Autodesk Fusion 360 part; units mm, degrees
(part 5 of 6)
  line L2682 (181.3394, 91.625) -> (181.127, 93.125)
  line L2683 (187.1203, 93.125) -> (188.1063, 86.1615)
  line L2684 (181.3454, 86.0752) -> (182.0837, 85.3126)
  line L2685 (180.927, 93.125) -> (181.8208, 86.8124)
  line L2686 (187.186, 86.0499) -> (186.4477, 86.8126)
  line L2687 (186.4603, 87.0871) -> (185.6054, 93.125)
  line L2688 (181.127, 93.125) -> (185.4054, 93.125)
  line L2689 (186.4477, 86.8126) -> (182.1089, 86.8126)
  line L2690 (185.6054, 93.125) -> (187.1203, 93.125)
  line L2691 (181.8208, 86.8124) -> (181.1478, 86.1625)
  line L2692 (198.3258, 91.625) -> (194.0474, 91.625)
  line L2693 (193.635, 93.125) -> (192.12, 93.125)
  arc A395 (201.2525, 79) -> (201.7476, 79.5701) centre (201.2525, 79.5) ccw
  circle A396 centre (192.12, 79.875) radius 0.875
  line L2694 (193.8842, 85.9625) -> (194.7802, 85.0369)
  line L2695 (200.3283, 79) -> (201.8283, 79)
  line L2696 (199.9139, 80.5) -> (195.6246, 80.5)
  line L2697 (194.8169, 86.8126) -> (194.0534, 86.0752)
  line L2698 (195.635, 79) -> (194.12, 79)
  line L2699 (194.12, 79) -> (193.1342, 85.9625)
  line L2700 (199.4326, 85.3263) -> (200.3283, 79)
  line L2701 (200.1263, 79) -> (199.9139, 80.5)
  line L2702 (199.1304, 85.3126) -> (199.894, 86.0499)
  line L2703 (200.8143, 86.1615) -> (200.0643, 86.1615)
  line L2704 (201.8283, 79) -> (200.8424, 85.9635)
  arc A397 (192.6958, 93.125) -> (192.2007, 92.5549) centre (192.6958, 92.625) ccw
  line L2705 (195.837, 79) -> (200.1263, 79)
  line L2706 (194.7802, 85.0369) -> (195.635, 79)
  line L2707 (200.0924, 85.9635) -> (199.4326, 85.3263)
  line L2708 (195.6246, 80.5) -> (195.837, 79)
  line L2709 (194.7917, 85.3126) -> (199.1304, 85.3126)
  line L2710 (200.0643, 86.1615) -> (199.1683, 87.0871)
  line L2711 (193.1342, 85.9625) -> (193.8842, 85.9625)
  line L2712 (200.8424, 85.9635) -> (200.0924, 85.9635)
  arc A398 (194.0591, 79.4299) -> (194.5542, 79) centre (194.5542, 79.5) ccw
  line L2713 (193.8558, 86.1625) -> (193.1058, 86.1625)
  line L2714 (198.1134, 93.125) -> (198.3258, 91.625)
  arc A399 (199.8892, 92.6951) -> (199.3941, 93.125) centre (199.3941, 92.625) ccw
  line L2715 (193.1058, 86.1625) -> (192.12, 93.125)
  line L2716 (194.0474, 91.625) -> (193.835, 93.125)
  line L2717 (199.8283, 93.125) -> (200.8143, 86.1615)
  line L2718 (194.0534, 86.0752) -> (194.7917, 85.3126)
  line L2719 (193.635, 93.125) -> (194.5288, 86.8124)
  line L2720 (199.894, 86.0499) -> (199.1557, 86.8126)
  line L2721 (199.1683, 87.0871) -> (198.3134, 93.125)
  line L2722 (193.835, 93.125) -> (198.1134, 93.125)
  line L2723 (199.1557, 86.8126) -> (194.8169, 86.8126)
  line L2724 (198.3134, 93.125) -> (199.8283, 93.125)
  line L2725 (194.5288, 86.8124) -> (193.8558, 86.1625)
  line L2726 (7.7058, 110.75) -> (3.4274, 110.75)
  line L2727 (3.015, 112.25) -> (1.5, 112.25)
  arc A400 (10.6325, 98.125) -> (11.1276, 98.6951) centre (10.6325, 98.625) ccw
  circle A401 centre (1.5, 99) radius 0.875
  line L2728 (3.2642, 105.0875) -> (4.1602, 104.1619)
  line L2729 (9.7083, 98.125) -> (11.2083, 98.125)
  line L2730 (9.2939, 99.625) -> (5.0046, 99.625)
  line L2731 (4.1969, 105.9376) -> (3.4334, 105.2002)
  line L2732 (5.015, 98.125) -> (3.5, 98.125)
  line L2733 (3.5, 98.125) -> (2.5142, 105.0875)
  line L2734 (8.8126, 104.4513) -> (9.7083, 98.125)
  line L2735 (9.5063, 98.125) -> (9.2939, 99.625)
  line L2736 (8.5104, 104.4376) -> (9.274, 105.1749)
  line L2737 (10.1943, 105.2865) -> (9.4443, 105.2865)
  line L2738 (11.2083, 98.125) -> (10.2224, 105.0885)
  arc A402 (2.0758, 112.25) -> (1.5807, 111.6799) centre (2.0758, 111.75) ccw
  line L2739 (5.217, 98.125) -> (9.5063, 98.125)
  line L2740 (4.1602, 104.1619) -> (5.015, 98.125)
  line L2741 (9.4724, 105.0885) -> (8.8126, 104.4513)
  line L2742 (5.0046, 99.625) -> (5.217, 98.125)
  line L2743 (4.1717, 104.4376) -> (8.5104, 104.4376)
  line L2744 (9.4443, 105.2865) -> (8.5483, 106.2121)
  line L2745 (2.5142, 105.0875) -> (3.2642, 105.0875)
  line L2746 (10.2224, 105.0885) -> (9.4724, 105.0885)
  arc A403 (3.4391, 98.5549) -> (3.9342, 98.125) centre (3.9342, 98.625) ccw
  line L2747 (3.2358, 105.2875) -> (2.4858, 105.2875)
  line L2748 (7.4934, 112.25) -> (7.7058, 110.75)
  arc A404 (9.2692, 111.8201) -> (8.7741, 112.25) centre (8.7741, 111.75) ccw
  line L2749 (2.4858, 105.2875) -> (1.5, 112.25)
  line L2750 (3.4274, 110.75) -> (3.215, 112.25)
  line L2751 (9.2083, 112.25) -> (10.1943, 105.2865)
  line L2752 (3.4334, 105.2002) -> (4.1717, 104.4376)
  line L2753 (3.015, 112.25) -> (3.9088, 105.9374)
  line L2754 (9.274, 105.1749) -> (8.5357, 105.9376)
  line L2755 (8.5483, 106.2121) -> (7.6934, 112.25)
  line L2756 (3.215, 112.25) -> (7.4934, 112.25)
  line L2757 (8.5357, 105.9376) -> (4.1969, 105.9376)
  line L2758 (7.6934, 112.25) -> (9.2083, 112.25)
  line L2759 (3.9088, 105.9374) -> (3.2358, 105.2875)
  line L2760 (20.4138, 110.75) -> (16.1354, 110.75)
  line L2761 (15.723, 112.25) -> (14.208, 112.25)
  arc A405 (23.3405, 98.125) -> (23.8356, 98.6951) centre (23.3405, 98.625) ccw
  circle A406 centre (14.208, 99) radius 0.875
  line L2762 (15.9722, 105.0875) -> (16.8682, 104.1619)
  line L2763 (22.4163, 98.125) -> (23.9163, 98.125)
  line L2764 (22.0019, 99.625) -> (17.7126, 99.625)
  line L2765 (16.9049, 105.9376) -> (16.1414, 105.2002)
  line L2766 (17.723, 98.125) -> (16.208, 98.125)
  line L2767 (16.208, 98.125) -> (15.2222, 105.0875)
  line L2768 (21.5206, 104.4513) -> (22.4163, 98.125)
  line L2769 (22.2143, 98.125) -> (22.0019, 99.625)
  line L2770 (21.2184, 104.4376) -> (21.982, 105.1749)
  line L2771 (22.9023, 105.2865) -> (22.1523, 105.2865)
  line L2772 (23.9163, 98.125) -> (22.9304, 105.0885)
  arc A407 (14.7838, 112.25) -> (14.2887, 111.6799) centre (14.7838, 111.75) ccw
  line L2773 (17.925, 98.125) -> (22.2143, 98.125)
  line L2774 (16.8682, 104.1619) -> (17.723, 98.125)
  line L2775 (22.1804, 105.0885) -> (21.5206, 104.4513)
  line L2776 (17.7126, 99.625) -> (17.925, 98.125)
  line L2777 (16.8797, 104.4376) -> (21.2184, 104.4376)
  line L2778 (22.1523, 105.2865) -> (21.2563, 106.2121)
  line L2779 (15.2222, 105.0875) -> (15.9722, 105.0875)
  line L2780 (22.9304, 105.0885) -> (22.1804, 105.0885)
  arc A408 (16.1471, 98.5549) -> (16.6422, 98.125) centre (16.6422, 98.625) ccw
  line L2781 (15.9438, 105.2875) -> (15.1938, 105.2875)
  line L2782 (20.2014, 112.25) -> (20.4138, 110.75)
  arc A409 (21.9772, 111.8201) -> (21.4821, 112.25) centre (21.4821, 111.75) ccw
  line L2783 (15.1938, 105.2875) -> (14.208, 112.25)
  line L2784 (16.1354, 110.75) -> (15.923, 112.25)
  line L2785 (21.9163, 112.25) -> (22.9023, 105.2865)
  line L2786 (16.1414, 105.2002) -> (16.8797, 104.4376)
  line L2787 (15.723, 112.25) -> (16.6168, 105.9374)
  line L2788 (21.982, 105.1749) -> (21.2437, 105.9376)
  line L2789 (21.2563, 106.2121) -> (20.4014, 112.25)
  line L2790 (15.923, 112.25) -> (20.2014, 112.25)
  line L2791 (21.2437, 105.9376) -> (16.9049, 105.9376)
  line L2792 (20.4014, 112.25) -> (21.9163, 112.25)
  line L2793 (16.6168, 105.9374) -> (15.9438, 105.2875)
  line L2794 (33.1218, 110.75) -> (28.8434, 110.75)
  line L2795 (28.431, 112.25) -> (26.916, 112.25)
  arc A410 (36.0485, 98.125) -> (36.5436, 98.6951) centre (36.0485, 98.625) ccw
  circle A411 centre (26.916, 99) radius 0.875
  line L2796 (28.6802, 105.0875) -> (29.5762, 104.1619)
  line L2797 (35.1243, 98.125) -> (36.6243, 98.125)
  line L2798 (34.7099, 99.625) -> (30.4206, 99.625)
  line L2799 (29.6129, 105.9376) -> (28.8494, 105.2002)
  line L2800 (30.431, 98.125) -> (28.916, 98.125)
  line L2801 (28.916, 98.125) -> (27.9302, 105.0875)
  line L2802 (34.2286, 104.4513) -> (35.1243, 98.125)
  line L2803 (34.9223, 98.125) -> (34.7099, 99.625)
  line L2804 (33.9264, 104.4376) -> (34.69, 105.1749)
  line L2805 (35.6103, 105.2865) -> (34.8603, 105.2865)
  line L2806 (36.6243, 98.125) -> (35.6384, 105.0885)
  arc A412 (27.4918, 112.25) -> (26.9967, 111.6799) centre (27.4918, 111.75) ccw
  line L2807 (30.633, 98.125) -> (34.9223, 98.125)
  line L2808 (29.5762, 104.1619) -> (30.431, 98.125)
  line L2809 (34.8884, 105.0885) -> (34.2286, 104.4513)
  line L2810 (30.4206, 99.625) -> (30.633, 98.125)
  line L2811 (29.5877, 104.4376) -> (33.9264, 104.4376)
  line L2812 (34.8603, 105.2865) -> (33.9643, 106.2121)
  line L2813 (27.9302, 105.0875) -> (28.6802, 105.0875)
  line L2814 (35.6384, 105.0885) -> (34.8884, 105.0885)
  arc A413 (28.8551, 98.5549) -> (29.3502, 98.125) centre (29.3502, 98.625) ccw
  line L2815 (28.6518, 105.2875) -> (27.9018, 105.2875)
  line L2816 (32.9094, 112.25) -> (33.1218, 110.75)
  arc A414 (34.6852, 111.8201) -> (34.1901, 112.25) centre (34.1901, 111.75) ccw
  line L2817 (27.9018, 105.2875) -> (26.916, 112.25)
  line L2818 (28.8434, 110.75) -> (28.631, 112.25)
  line L2819 (34.6243, 112.25) -> (35.6103, 105.2865)
  line L2820 (28.8494, 105.2002) -> (29.5877, 104.4376)
  line L2821 (28.431, 112.25) -> (29.3248, 105.9374)
  line L2822 (34.69, 105.1749) -> (33.9517, 105.9376)
  line L2823 (33.9643, 106.2121) -> (33.1094, 112.25)
  line L2824 (28.631, 112.25) -> (32.9094, 112.25)
  line L2825 (33.9517, 105.9376) -> (29.6129, 105.9376)
  line L2826 (33.1094, 112.25) -> (34.6243, 112.25)
  line L2827 (29.3248, 105.9374) -> (28.6518, 105.2875)
  line L2828 (45.8298, 110.75) -> (41.5514, 110.75)
  line L2829 (41.139, 112.25) -> (39.624, 112.25)
  arc A415 (48.7565, 98.125) -> (49.2516, 98.6951) centre (48.7565, 98.625) ccw
  circle A416 centre (39.624, 99) radius 0.875
  line L2830 (41.3882, 105.0875) -> (42.2842, 104.1619)
  line L2831 (47.8323, 98.125) -> (49.3323, 98.125)
  line L2832 (47.4179, 99.625) -> (43.1286, 99.625)
  line L2833 (42.3209, 105.9376) -> (41.5574, 105.2002)
  line L2834 (43.139, 98.125) -> (41.624, 98.125)
  line L2835 (41.624, 98.125) -> (40.6382, 105.0875)
  line L2836 (46.9366, 104.4513) -> (47.8323, 98.125)
  line L2837 (47.6303, 98.125) -> (47.4179, 99.625)
  line L2838 (46.6344, 104.4376) -> (47.398, 105.1749)
  line L2839 (48.3183, 105.2865) -> (47.5683, 105.2865)
  line L2840 (49.3323, 98.125) -> (48.3464, 105.0885)
  arc A417 (40.1998, 112.25) -> (39.7047, 111.6799) centre (40.1998, 111.75) ccw
  line L2841 (43.341, 98.125) -> (47.6303, 98.125)
  line L2842 (42.2842, 104.1619) -> (43.139, 98.125)
  line L2843 (47.5964, 105.0885) -> (46.9366, 104.4513)
  line L2844 (43.1286, 99.625) -> (43.341, 98.125)
  line L2845 (42.2957, 104.4376) -> (46.6344, 104.4376)
  line L2846 (47.5683, 105.2865) -> (46.6723, 106.2121)
  line L2847 (40.6382, 105.0875) -> (41.3882, 105.0875)
  line L2848 (48.3464, 105.0885) -> (47.5964, 105.0885)
  arc A418 (41.5631, 98.5549) -> (42.0582, 98.125) centre (42.0582, 98.625) ccw
  line L2849 (41.3598, 105.2875) -> (40.6098, 105.2875)
  line L2850 (45.6174, 112.25) -> (45.8298, 110.75)
  arc A419 (47.3932, 111.8201) -> (46.8981, 112.25) centre (46.8981, 111.75) ccw
  line L2851 (40.6098, 105.2875) -> (39.624, 112.25)
  line L2852 (41.5514, 110.75) -> (41.339, 112.25)
  line L2853 (47.3323, 112.25) -> (48.3183, 105.2865)
  line L2854 (41.5574, 105.2002) -> (42.2957, 104.4376)
  line L2855 (41.139, 112.25) -> (42.0328, 105.9374)
  line L2856 (47.398, 105.1749) -> (46.6597, 105.9376)
  line L2857 (46.6723, 106.2121) -> (45.8174, 112.25)
  line L2858 (41.339, 112.25) -> (45.6174, 112.25)
  line L2859 (46.6597, 105.9376) -> (42.3209, 105.9376)
  line L2860 (45.8174, 112.25) -> (47.3323, 112.25)
  line L2861 (42.0328, 105.9374) -> (41.3598, 105.2875)
  line L2862 (58.5378, 110.75) -> (54.2594, 110.75)
  line L2863 (53.847, 112.25) -> (52.332, 112.25)
  arc A420 (61.4645, 98.125) -> (61.9596, 98.6951) centre (61.4645, 98.625) ccw
  circle A421 centre (52.332, 99) radius 0.875
  line L2864 (54.0962, 105.0875) -> (54.9922, 104.1619)
  line L2865 (60.5403, 98.125) -> (62.0403, 98.125)
  line L2866 (60.1259, 99.625) -> (55.8366, 99.625)
  line L2867 (55.0289, 105.9376) -> (54.2654, 105.2002)
  line L2868 (55.847, 98.125) -> (54.332, 98.125)
  line L2869 (54.332, 98.125) -> (53.3462, 105.0875)
  line L2870 (59.6446, 104.4513) -> (60.5403, 98.125)
  line L2871 (60.3383, 98.125) -> (60.1259, 99.625)
  line L2872 (59.3424, 104.4376) -> (60.106, 105.1749)
  line L2873 (61.0263, 105.2865) -> (60.2763, 105.2865)
  line L2874 (62.0403, 98.125) -> (61.0544, 105.0885)
  arc A422 (52.9078, 112.25) -> (52.4127, 111.6799) centre (52.9078, 111.75) ccw
  line L2875 (56.049, 98.125) -> (60.3383, 98.125)
  line L2876 (54.9922, 104.1619) -> (55.847, 98.125)
  line L2877 (60.3044, 105.0885) -> (59.6446, 104.4513)
  line L2878 (55.8366, 99.625) -> (56.049, 98.125)
  line L2879 (55.0037, 104.4376) -> (59.3424, 104.4376)
  line L2880 (60.2763, 105.2865) -> (59.3803, 106.2121)
  line L2881 (53.3462, 105.0875) -> (54.0962, 105.0875)
  line L2882 (61.0544, 105.0885) -> (60.3044, 105.0885)
  arc A423 (54.2711, 98.5549) -> (54.7662, 98.125) centre (54.7662, 98.625) ccw
  line L2883 (54.0678, 105.2875) -> (53.3178, 105.2875)
  line L2884 (58.3254, 112.25) -> (58.5378, 110.75)
  arc A424 (60.1012, 111.8201) -> (59.6061, 112.25) centre (59.6061, 111.75) ccw
  line L2885 (53.3178, 105.2875) -> (52.332, 112.25)
  line L2886 (54.2594, 110.75) -> (54.047, 112.25)
  line L2887 (60.0403, 112.25) -> (61.0263, 105.2865)
  line L2888 (54.2654, 105.2002) -> (55.0037, 104.4376)
  line L2889 (53.847, 112.25) -> (54.7408, 105.9374)
  line L2890 (60.106, 105.1749) -> (59.3677, 105.9376)
  line L2891 (59.3803, 106.2121) -> (58.5254, 112.25)
  line L2892 (54.047, 112.25) -> (58.3254, 112.25)
  line L2893 (59.3677, 105.9376) -> (55.0289, 105.9376)
  line L2894 (58.5254, 112.25) -> (60.0403, 112.25)
  line L2895 (54.7408, 105.9374) -> (54.0678, 105.2875)
  line L2896 (71.2458, 110.75) -> (66.9674, 110.75)
  line L2897 (66.555, 112.25) -> (65.04, 112.25)
  arc A425 (74.1725, 98.125) -> (74.6676, 98.6951) centre (74.1725, 98.625) ccw
  circle A426 centre (65.04, 99) radius 0.875
  line L2898 (66.8042, 105.0875) -> (67.7002, 104.1619)
  line L2899 (73.2483, 98.125) -> (74.7483, 98.125)
  line L2900 (72.8339, 99.625) -> (68.5446, 99.625)
  line L2901 (67.7369, 105.9376) -> (66.9734, 105.2002)
  line L2902 (68.555, 98.125) -> (67.04, 98.125)
  line L2903 (67.04, 98.125) -> (66.0542, 105.0875)
  line L2904 (72.3526, 104.4513) -> (73.2483, 98.125)
  line L2905 (73.0463, 98.125) -> (72.8339, 99.625)
  line L2906 (72.0504, 104.4376) -> (72.814, 105.1749)
  line L2907 (73.7343, 105.2865) -> (72.9843, 105.2865)
  line L2908 (74.7483, 98.125) -> (73.7624, 105.0885)
  arc A427 (65.6158, 112.25) -> (65.1207, 111.6799) centre (65.6158, 111.75) ccw
  line L2909 (68.757, 98.125) -> (73.0463, 98.125)
  line L2910 (67.7002, 104.1619) -> (68.555, 98.125)
  line L2911 (73.0124, 105.0885) -> (72.3526, 104.4513)
  line L2912 (68.5446, 99.625) -> (68.757, 98.125)
  line L2913 (67.7117, 104.4376) -> (72.0504, 104.4376)
  line L2914 (72.9843, 105.2865) -> (72.0883, 106.2121)
  line L2915 (66.0542, 105.0875) -> (66.8042, 105.0875)
  line L2916 (73.7624, 105.0885) -> (73.0124, 105.0885)
  arc A428 (66.9791, 98.5549) -> (67.4742, 98.125) centre (67.4742, 98.625) ccw
  line L2917 (66.7758, 105.2875) -> (66.0258, 105.2875)
  line L2918 (71.0334, 112.25) -> (71.2458, 110.75)
  arc A429 (72.8092, 111.8201) -> (72.3141, 112.25) centre (72.3141, 111.75) ccw
  line L2919 (66.0258, 105.2875) -> (65.04, 112.25)
  line L2920 (66.9674, 110.75) -> (66.755, 112.25)
  line L2921 (72.7483, 112.25) -> (73.7343, 105.2865)
  line L2922 (66.9734, 105.2002) -> (67.7117, 104.4376)
  line L2923 (66.555, 112.25) -> (67.4488, 105.9374)
  line L2924 (72.814, 105.1749) -> (72.0757, 105.9376)
  line L2925 (72.0883, 106.2121) -> (71.2334, 112.25)
  line L2926 (66.755, 112.25) -> (71.0334, 112.25)
  line L2927 (72.0757, 105.9376) -> (67.7369, 105.9376)
  line L2928 (71.2334, 112.25) -> (72.7483, 112.25)
  line L2929 (67.4488, 105.9374) -> (66.7758, 105.2875)
  line L2930 (83.9538, 110.75) -> (79.6754, 110.75)
  line L2931 (79.263, 112.25) -> (77.748, 112.25)
  arc A430 (86.8805, 98.125) -> (87.3756, 98.6951) centre (86.8805, 98.625) ccw
  circle A431 centre (77.748, 99) radius 0.875
  line L2932 (79.5122, 105.0875) -> (80.4082, 104.1619)
  line L2933 (85.9563, 98.125) -> (87.4563, 98.125)
  line L2934 (85.5419, 99.625) -> (81.2526, 99.625)
  line L2935 (80.4449, 105.9376) -> (79.6814, 105.2002)
  line L2936 (81.263, 98.125) -> (79.748, 98.125)
  line L2937 (79.748, 98.125) -> (78.7622, 105.0875)
  line L2938 (85.0606, 104.4513) -> (85.9563, 98.125)
  line L2939 (85.7543, 98.125) -> (85.5419, 99.625)
  line L2940 (84.7584, 104.4376) -> (85.522, 105.1749)
  line L2941 (86.4423, 105.2865) -> (85.6923, 105.2865)
  line L2942 (87.4563, 98.125) -> (86.4704, 105.0885)
  arc A432 (78.3238, 112.25) -> (77.8287, 111.6799) centre (78.3238, 111.75) ccw
  line L2943 (81.465, 98.125) -> (85.7543, 98.125)
  line L2944 (80.4082, 104.1619) -> (81.263, 98.125)
  line L2945 (85.7204, 105.0885) -> (85.0606, 104.4513)
  line L2946 (81.2526, 99.625) -> (81.465, 98.125)
  line L2947 (80.4197, 104.4376) -> (84.7584, 104.4376)
  line L2948 (85.6923, 105.2865) -> (84.7963, 106.2121)
  line L2949 (78.7622, 105.0875) -> (79.5122, 105.0875)
  line L2950 (86.4704, 105.0885) -> (85.7204, 105.0885)
  arc A433 (79.6871, 98.5549) -> (80.1822, 98.125) centre (80.1822, 98.625) ccw
  line L2951 (79.4838, 105.2875) -> (78.7338, 105.2875)
  line L2952 (83.7414, 112.25) -> (83.9538, 110.75)
  arc A434 (85.5172, 111.8201) -> (85.0221, 112.25) centre (85.0221, 111.75) ccw
  line L2953 (78.7338, 105.2875) -> (77.748, 112.25)
  line L2954 (79.6754, 110.75) -> (79.463, 112.25)
  line L2955 (85.4563, 112.25) -> (86.4423, 105.2865)
  line L2956 (79.6814, 105.2002) -> (80.4197, 104.4376)
  line L2957 (79.263, 112.25) -> (80.1568, 105.9374)
  line L2958 (85.522, 105.1749) -> (84.7837, 105.9376)
  line L2959 (84.7963, 106.2121) -> (83.9414, 112.25)
  line L2960 (79.463, 112.25) -> (83.7414, 112.25)
  line L2961 (84.7837, 105.9376) -> (80.4449, 105.9376)
  line L2962 (83.9414, 112.25) -> (85.4563, 112.25)
  line L2963 (80.1568, 105.9374) -> (79.4838, 105.2875)
  line L2964 (96.6618, 110.75) -> (92.3834, 110.75)
  line L2965 (91.971, 112.25) -> (90.456, 112.25)
  arc A435 (99.5885, 98.125) -> (100.0836, 98.6951) centre (99.5885, 98.625) ccw
  circle A436 centre (90.456, 99) radius 0.875
  line L2966 (92.2202, 105.0875) -> (93.1162, 104.1619)
  line L2967 (98.6643, 98.125) -> (100.1643, 98.125)
  line L2968 (98.2499, 99.625) -> (93.9606, 99.625)
  line L2969 (93.1529, 105.9376) -> (92.3894, 105.2002)
  line L2970 (93.971, 98.125) -> (92.456, 98.125)
  line L2971 (92.456, 98.125) -> (91.4702, 105.0875)
  line L2972 (97.7686, 104.4513) -> (98.6643, 98.125)
  line L2973 (98.4623, 98.125) -> (98.2499, 99.625)
  line L2974 (97.4664, 104.4376) -> (98.23, 105.1749)
  line L2975 (99.1503, 105.2865) -> (98.4003, 105.2865)
  line L2976 (100.1643, 98.125) -> (99.1784, 105.0885)
  arc A437 (91.0318, 112.25) -> (90.5367, 111.6799) centre (91.0318, 111.75) ccw
  line L2977 (94.173, 98.125) -> (98.4623, 98.125)
  line L2978 (93.1162, 104.1619) -> (93.971, 98.125)
  line L2979 (98.4284, 105.0885) -> (97.7686, 104.4513)
  line L2980 (93.9606, 99.625) -> (94.173, 98.125)
  line L2981 (93.1277, 104.4376) -> (97.4664, 104.4376)
  line L2982 (98.4003, 105.2865) -> (97.5043, 106.2121)
  line L2983 (91.4702, 105.0875) -> (92.2202, 105.0875)
  line L2984 (99.1784, 105.0885) -> (98.4284, 105.0885)
  arc A438 (92.3951, 98.5549) -> (92.8902, 98.125) centre (92.8902, 98.625) ccw
  line L2985 (92.1918, 105.2875) -> (91.4418, 105.2875)
  line L2986 (96.4494, 112.25) -> (96.6618, 110.75)
  arc A439 (98.2252, 111.8201) -> (97.7301, 112.25) centre (97.7301, 111.75) ccw
  line L2987 (91.4418, 105.2875) -> (90.456, 112.25)
  line L2988 (92.3834, 110.75) -> (92.171, 112.25)
  line L2989 (98.1643, 112.25) -> (99.1503, 105.2865)
  line L2990 (92.3894, 105.2002) -> (93.1277, 104.4376)
  line L2991 (91.971, 112.25) -> (92.8648, 105.9374)
  line L2992 (98.23, 105.1749) -> (97.4917, 105.9376)
  line L2993 (97.5043, 106.2121) -> (96.6494, 112.25)
  line L2994 (92.171, 112.25) -> (96.4494, 112.25)
  line L2995 (97.4917, 105.9376) -> (93.1529, 105.9376)
  line L2996 (96.6494, 112.25) -> (98.1643, 112.25)
  line L2997 (92.8648, 105.9374) -> (92.1918, 105.2875)
  line L2998 (109.3698, 110.75) -> (105.0914, 110.75)
  line L2999 (104.679, 112.25) -> (103.164, 112.25)
  arc A440 (112.2965, 98.125) -> (112.7916, 98.6951) centre (112.2965, 98.625) ccw
  circle A441 centre (103.164, 99) radius 0.875
  line L3000 (104.9282, 105.0875) -> (105.8242, 104.1619)
  line L3001 (111.3723, 98.125) -> (112.8723, 98.125)
  line L3002 (110.9579, 99.625) -> (106.6686, 99.625)
  line L3003 (105.8609, 105.9376) -> (105.0974, 105.2002)
  line L3004 (106.679, 98.125) -> (105.164, 98.125)
  line L3005 (105.164, 98.125) -> (104.1782, 105.0875)
  line L3006 (110.4766, 104.4513) -> (111.3723, 98.125)
  line L3007 (111.1703, 98.125) -> (110.9579, 99.625)
  line L3008 (110.1744, 104.4376) -> (110.938, 105.1749)
  line L3009 (111.8583, 105.2865) -> (111.1083, 105.2865)
  line L3010 (112.8723, 98.125) -> (111.8864, 105.0885)
  arc A442 (103.7398, 112.25) -> (103.2447, 111.6799) centre (103.7398, 111.75) ccw
  line L3011 (106.881, 98.125) -> (111.1703, 98.125)
  line L3012 (105.8242, 104.1619) -> (106.679, 98.125)
  line L3013 (111.1364, 105.0885) -> (110.4766, 104.4513)
  line L3014 (106.6686, 99.625) -> (106.881, 98.125)
  line L3015 (105.8357, 104.4376) -> (110.1744, 104.4376)
  line L3016 (111.1083, 105.2865) -> (110.2123, 106.2121)
  line L3017 (104.1782, 105.0875) -> (104.9282, 105.0875)
  line L3018 (111.8864, 105.0885) -> (111.1364, 105.0885)
  arc A443 (105.1031, 98.5549) -> (105.5982, 98.125) centre (105.5982, 98.625) ccw
  line L3019 (104.8998, 105.2875) -> (104.1498, 105.2875)
  line L3020 (109.1574, 112.25) -> (109.3698, 110.75)
  arc A444 (110.9332, 111.8201) -> (110.4381, 112.25) centre (110.4381, 111.75) ccw
  line L3021 (104.1498, 105.2875) -> (103.164, 112.25)
  line L3022 (105.0914, 110.75) -> (104.879, 112.25)
  line L3023 (110.8723, 112.25) -> (111.8583, 105.2865)
  line L3024 (105.0974, 105.2002) -> (105.8357, 104.4376)
  line L3025 (104.679, 112.25) -> (105.5728, 105.9374)
  line L3026 (110.938, 105.1749) -> (110.1997, 105.9376)
  line L3027 (110.2123, 106.2121) -> (109.3574, 112.25)
  line L3028 (104.879, 112.25) -> (109.1574, 112.25)
  line L3029 (110.1997, 105.9376) -> (105.8609, 105.9376)
  line L3030 (109.3574, 112.25) -> (110.8723, 112.25)
  line L3031 (105.5728, 105.9374) -> (104.8998, 105.2875)
  line L3032 (122.0778, 110.75) -> (117.7994, 110.75)
  line L3033 (117.387, 112.25) -> (115.872, 112.25)
  arc A445 (125.0045, 98.125) -> (125.4996, 98.6951) centre (125.0045, 98.625) ccw
  circle A446 centre (115.872, 99) radius 0.875
  line L3034 (117.6362, 105.0875) -> (118.5322, 104.1619)
  line L3035 (124.0803, 98.125) -> (125.5803, 98.125)
  line L3036 (123.6659, 99.625) -> (119.3766, 99.625)
  line L3037 (118.5689, 105.9376) -> (117.8054, 105.2002)
  line L3038 (119.387, 98.125) -> (117.872, 98.125)
  line L3039 (117.872, 98.125) -> (116.8862, 105.0875)
  line L3040 (123.1846, 104.4513) -> (124.0803, 98.125)
  line L3041 (123.8783, 98.125) -> (123.6659, 99.625)
  line L3042 (122.8824, 104.4376) -> (123.646, 105.1749)
  line L3043 (124.5663, 105.2865) -> (123.8163, 105.2865)
  line L3044 (125.5803, 98.125) -> (124.5944, 105.0885)
  arc A447 (116.4478, 112.25) -> (115.9527, 111.6799) centre (116.4478, 111.75) ccw
  line L3045 (119.589, 98.125) -> (123.8783, 98.125)
  line L3046 (118.5322, 104.1619) -> (119.387, 98.125)
  line L3047 (123.8444, 105.0885) -> (123.1846, 104.4513)
  line L3048 (119.3766, 99.625) -> (119.589, 98.125)
  line L3049 (118.5437, 104.4376) -> (122.8824, 104.4376)
  line L3050 (123.8163, 105.2865) -> (122.9203, 106.2121)
  line L3051 (116.8862, 105.0875) -> (117.6362, 105.0875)
  line L3052 (124.5944, 105.0885) -> (123.8444, 105.0885)
  arc A448 (117.8111, 98.5549) -> (118.3062, 98.125) centre (118.3062, 98.625) ccw
  line L3053 (117.6078, 105.2875) -> (116.8578, 105.2875)
  line L3054 (121.8654, 112.25) -> (122.0778, 110.75)
  arc A449 (123.6412, 111.8201) -> (123.1461, 112.25) centre (123.1461, 111.75) ccw
  line L3055 (116.8578, 105.2875) -> (115.872, 112.25)
  line L3056 (117.7994, 110.75) -> (117.587, 112.25)
  line L3057 (123.5803, 112.25) -> (124.5663, 105.2865)
  line L3058 (117.8054, 105.2002) -> (118.5437, 104.4376)
  line L3059 (117.387, 112.25) -> (118.2808, 105.9374)
  line L3060 (123.646, 105.1749) -> (122.9077, 105.9376)
  line L3061 (122.9203, 106.2121) -> (122.0654, 112.25)
  line L3062 (117.587, 112.25) -> (121.8654, 112.25)
  line L3063 (122.9077, 105.9376) -> (118.5689, 105.9376)
  line L3064 (122.0654, 112.25) -> (123.5803, 112.25)
  line L3065 (118.2808, 105.9374) -> (117.6078, 105.2875)
  line L3066 (134.7858, 110.75) -> (130.5074, 110.75)
  line L3067 (130.095, 112.25) -> (128.58, 112.25)
  arc A450 (137.7125, 98.125) -> (138.2076, 98.6951) centre (137.7125, 98.625) ccw
  circle A451 centre (128.58, 99) radius 0.875
  line L3068 (130.3442, 105.0875) -> (131.2402, 104.1619)
  line L3069 (136.7883, 98.125) -> (138.2883, 98.125)
  line L3070 (136.3739, 99.625) -> (132.0846, 99.625)
  line L3071 (131.2769, 105.9376) -> (130.5134, 105.2002)
  line L3072 (132.095, 98.125) -> (130.58, 98.125)
  line L3073 (130.58, 98.125) -> (129.5942, 105.0875)
  line L3074 (135.8926, 104.4513) -> (136.7883, 98.125)
  line L3075 (136.5863, 98.125) -> (136.3739, 99.625)
  line L3076 (135.5904, 104.4376) -> (136.354, 105.1749)
  line L3077 (137.2743, 105.2865) -> (136.5243, 105.2865)
  line L3078 (138.2883, 98.125) -> (137.3024, 105.0885)
  arc A452 (129.1558, 112.25) -> (128.6607, 111.6799) centre (129.1558, 111.75) ccw
  line L3079 (132.297, 98.125) -> (136.5863, 98.125)
  line L3080 (131.2402, 104.1619) -> (132.095, 98.125)
  line L3081 (136.5524, 105.0885) -> (135.8926, 104.4513)
  line L3082 (132.0846, 99.625) -> (132.297, 98.125)
  line L3083 (131.2517, 104.4376) -> (135.5904, 104.4376)
  line L3084 (136.5243, 105.2865) -> (135.6283, 106.2121)
  line L3085 (129.5942, 105.0875) -> (130.3442, 105.0875)
  line L3086 (137.3024, 105.0885) -> (136.5524, 105.0885)
  arc A453 (130.5191, 98.5549) -> (131.0142, 98.125) centre (131.0142, 98.625) ccw
  line L3087 (130.3158, 105.2875) -> (129.5658, 105.2875)
  line L3088 (134.5734, 112.25) -> (134.7858, 110.75)
  arc A454 (136.3492, 111.8201) -> (135.8541, 112.25) centre (135.8541, 111.75) ccw
  line L3089 (129.5658, 105.2875) -> (128.58, 112.25)
  line L3090 (130.5074, 110.75) -> (130.295, 112.25)
  line L3091 (136.2883, 112.25) -> (137.2743, 105.2865)
  line L3092 (130.5134, 105.2002) -> (131.2517, 104.4376)
  line L3093 (130.095, 112.25) -> (130.9888, 105.9374)
  line L3094 (136.354, 105.1749) -> (135.6157, 105.9376)
  line L3095 (135.6283, 106.2121) -> (134.7734, 112.25)
  line L3096 (130.295, 112.25) -> (134.5734, 112.25)
  line L3097 (135.6157, 105.9376) -> (131.2769, 105.9376)
  line L3098 (134.7734, 112.25) -> (136.2883, 112.25)
  line L3099 (130.9888, 105.9374) -> (130.3158, 105.2875)
  line L3100 (147.4938, 110.75) -> (143.2154, 110.75)
  line L3101 (142.803, 112.25) -> (141.288, 112.25)
  arc A455 (150.4205, 98.125) -> (150.9156, 98.6951) centre (150.4205, 98.625) ccw
  circle A456 centre (141.288, 99) radius 0.875
  line L3102 (143.0522, 105.0875) -> (143.9482, 104.1619)
  line L3103 (149.4963, 98.125) -> (150.9963, 98.125)
  line L3104 (149.0819, 99.625) -> (144.7926, 99.625)
  line L3105 (143.9849, 105.9376) -> (143.2214, 105.2002)
  line L3106 (144.803, 98.125) -> (143.288, 98.125)
  line L3107 (143.288, 98.125) -> (142.3022, 105.0875)
  line L3108 (148.6006, 104.4513) -> (149.4963, 98.125)
  line L3109 (149.2943, 98.125) -> (149.0819, 99.625)
  line L3110 (148.2984, 104.4376) -> (149.062, 105.1749)
  line L3111 (149.9823, 105.2865) -> (149.2323, 105.2865)
  line L3112 (150.9963, 98.125) -> (150.0104, 105.0885)
  arc A457 (141.8638, 112.25) -> (141.3687, 111.6799) centre (141.8638, 111.75) ccw
  line L3113 (145.005, 98.125) -> (149.2943, 98.125)
  line L3114 (143.9482, 104.1619) -> (144.803, 98.125)
  line L3115 (149.2604, 105.0885) -> (148.6006, 104.4513)
  line L3116 (144.7926, 99.625) -> (145.005, 98.125)
  line L3117 (143.9597, 104.4376) -> (148.2984, 104.4376)
  line L3118 (149.2323, 105.2865) -> (148.3363, 106.2121)
  line L3119 (142.3022, 105.0875) -> (143.0522, 105.0875)
  line L3120 (150.0104, 105.0885) -> (149.2604, 105.0885)
  arc A458 (143.2271, 98.5549) -> (143.7222, 98.125) centre (143.7222, 98.625) ccw
  line L3121 (143.0238, 105.2875) -> (142.2738, 105.2875)
  line L3122 (147.2814, 112.25) -> (147.4938, 110.75)
  arc A459 (149.0572, 111.8201) -> (148.5621, 112.25) centre (148.5621, 111.75) ccw
  line L3123 (142.2738, 105.2875) -> (141.288, 112.25)
  line L3124 (143.2154, 110.75) -> (143.003, 112.25)
  line L3125 (148.9963, 112.25) -> (149.9823, 105.2865)
  line L3126 (143.2214, 105.2002) -> (143.9597, 104.4376)
  line L3127 (142.803, 112.25) -> (143.6968, 105.9374)
  line L3128 (149.062, 105.1749) -> (148.3237, 105.9376)
  line L3129 (148.3363, 106.2121) -> (147.4814, 112.25)
  line L3130 (143.003, 112.25) -> (147.2814, 112.25)
  line L3131 (148.3237, 105.9376) -> (143.9849, 105.9376)
  line L3132 (147.4814, 112.25) -> (148.9963, 112.25)
  line L3133 (143.6968, 105.9374) -> (143.0238, 105.2875)
  line L3134 (160.2018, 110.75) -> (155.9234, 110.75)
  line L3135 (155.511, 112.25) -> (153.996, 112.25)
  arc A460 (163.1285, 98.125) -> (163.6236, 98.6951) centre (163.1285, 98.625) ccw
  circle A461 centre (153.996, 99) radius 0.875
  line L3136 (155.7602, 105.0875) -> (156.6562, 104.1619)
  line L3137 (162.2043, 98.125) -> (163.7043, 98.125)
  line L3138 (161.7899, 99.625) -> (157.5006, 99.625)
  line L3139 (156.6929, 105.9376) -> (155.9294, 105.2002)
  line L3140 (157.511, 98.125) -> (155.996, 98.125)
  line L3141 (155.996, 98.125) -> (155.0102, 105.0875)
  line L3142 (161.3086, 104.4513) -> (162.2043, 98.125)
  line L3143 (162.0023, 98.125) -> (161.7899, 99.625)
  line L3144 (161.0064, 104.4376) -> (161.77, 105.1749)
  line L3145 (162.6903, 105.2865) -> (161.9403, 105.2865)
  line L3146 (163.7043, 98.125) -> (162.7184, 105.0885)
  arc A462 (154.5718, 112.25) -> (154.0767, 111.6799) centre (154.5718, 111.75) ccw
  line L3147 (157.713, 98.125) -> (162.0023, 98.125)
  line L3148 (156.6562, 104.1619) -> (157.511, 98.125)
  line L3149 (161.9684, 105.0885) -> (161.3086, 104.4513)
  line L3150 (157.5006, 99.625) -> (157.713, 98.125)
  line L3151 (156.6677, 104.4376) -> (161.0064, 104.4376)
  line L3152 (161.9403, 105.2865) -> (161.0443, 106.2121)
  line L3153 (155.0102, 105.0875) -> (155.7602, 105.0875)
  line L3154 (162.7184, 105.0885) -> (161.9684, 105.0885)
  arc A463 (155.9351, 98.5549) -> (156.4302, 98.125) centre (156.4302, 98.625) ccw
  line L3155 (155.7318, 105.2875) -> (154.9818, 105.2875)
  line L3156 (159.9894, 112.25) -> (160.2018, 110.75)
  arc A464 (161.7652, 111.8201) -> (161.2701, 112.25) centre (161.2701, 111.75) ccw
  line L3157 (154.9818, 105.2875) -> (153.996, 112.25)
  line L3158 (155.9234, 110.75) -> (155.711, 112.25)
  line L3159 (161.7043, 112.25) -> (162.6903, 105.2865)
  line L3160 (155.9294, 105.2002) -> (156.6677, 104.4376)
  line L3161 (155.511, 112.25) -> (156.4048, 105.9374)
  line L3162 (161.77, 105.1749) -> (161.0317, 105.9376)
  line L3163 (161.0443, 106.2121) -> (160.1894, 112.25)
  line L3164 (155.711, 112.25) -> (159.9894, 112.25)
  line L3165 (161.0317, 105.9376) -> (156.6929, 105.9376)
  line L3166 (160.1894, 112.25) -> (161.7043, 112.25)
  line L3167 (156.4048, 105.9374) -> (155.7318, 105.2875)
  line L3168 (172.9098, 110.75) -> (168.6314, 110.75)
  line L3169 (168.219, 112.25) -> (166.704, 112.25)
  arc A465 (175.8365, 98.125) -> (176.3316, 98.6951) centre (175.8365, 98.625) ccw
  circle A466 centre (166.704, 99) radius 0.875
  line L3170 (168.4682, 105.0875) -> (169.3642, 104.1619)
  line L3171 (174.9123, 98.125) -> (176.4123, 98.125)
  line L3172 (174.4979, 99.625) -> (170.2086, 99.625)
  line L3173 (169.4009, 105.9376) -> (168.6374, 105.2002)
  line L3174 (170.219, 98.125) -> (168.704, 98.125)
  line L3175 (168.704, 98.125) -> (167.7182, 105.0875)
  line L3176 (174.0166, 104.4513) -> (174.9123, 98.125)
  line L3177 (174.7103, 98.125) -> (174.4979, 99.625)
  line L3178 (173.7144, 104.4376) -> (174.478, 105.1749)
  line L3179 (175.3983, 105.2865) -> (174.6483, 105.2865)
  line L3180 (176.4123, 98.125) -> (175.4264, 105.0885)
  arc A467 (167.2798, 112.25) -> (166.7847, 111.6799) centre (167.2798, 111.75) ccw
  line L3181 (170.421, 98.125) -> (174.7103, 98.125)
  line L3182 (169.3642, 104.1619) -> (170.219, 98.125)
  line L3183 (174.6764, 105.0885) -> (174.0166, 104.4513)
  line L3184 (170.2086, 99.625) -> (170.421, 98.125)
  line L3185 (169.3757, 104.4376) -> (173.7144, 104.4376)
  line L3186 (174.6483, 105.2865) -> (173.7523, 106.2121)
  line L3187 (167.7182, 105.0875) -> (168.4682, 105.0875)
  line L3188 (175.4264, 105.0885) -> (174.6764, 105.0885)
  arc A468 (168.6431, 98.5549) -> (169.1382, 98.125) centre (169.1382, 98.625) ccw
  line L3189 (168.4398, 105.2875) -> (167.6898, 105.2875)
  line L3190 (172.6974, 112.25) -> (172.9098, 110.75)
  arc A469 (174.4732, 111.8201) -> (173.9781, 112.25) centre (173.9781, 111.75) ccw
  line L3191 (167.6898, 105.2875) -> (166.704, 112.25)
  line L3192 (168.6314, 110.75) -> (168.419, 112.25)
  line L3193 (174.4123, 112.25) -> (175.3983, 105.2865)
  line L3194 (168.6374, 105.2002) -> (169.3757, 104.4376)
  line L3195 (168.219, 112.25) -> (169.1128, 105.9374)
  line L3196 (174.478, 105.1749) -> (173.7397, 105.9376)
  line L3197 (173.7523, 106.2121) -> (172.8974, 112.25)
  line L3198 (168.419, 112.25) -> (172.6974, 112.25)
  line L3199 (173.7397, 105.9376) -> (169.4009, 105.9376)
  line L3200 (172.8974, 112.25) -> (174.4123, 112.25)
  line L3201 (169.1128, 105.9374) -> (168.4398, 105.2875)
  line L3202 (185.6178, 110.75) -> (181.3394, 110.75)
  line L3203 (180.927, 112.25) -> (179.412, 112.25)
  arc A470 (188.5445, 98.125) -> (189.0396, 98.6951) centre (188.5445, 98.625) ccw
  circle A471 centre (179.412, 99) radius 0.875
  line L3204 (181.1762, 105.0875) -> (182.0722, 104.1619)
  line L3205 (187.6203, 98.125) -> (189.1203, 98.125)
  line L3206 (187.2059, 99.625) -> (182.9166, 99.625)
  line L3207 (182.1089, 105.9376) -> (181.3454, 105.2002)
  line L3208 (182.927, 98.125) -> (181.412, 98.125)
  line L3209 (181.412, 98.125) -> (180.4262, 105.0875)
  line L3210 (186.7246, 104.4513) -> (187.6203, 98.125)
  line L3211 (187.4183, 98.125) -> (187.2059, 99.625)
  line L3212 (186.4224, 104.4376) -> (187.186, 105.1749)
  line L3213 (188.1063, 105.2865) -> (187.3563, 105.2865)
  line L3214 (189.1203, 98.125) -> (188.1344, 105.0885)
  arc A472 (179.9878, 112.25) -> (179.4927, 111.6799) centre (179.9878, 111.75) ccw
  line L3215 (183.129, 98.125) -> (187.4183, 98.125)
  line L3216 (182.0722, 104.1619) -> (182.927, 98.125)
  line L3217 (187.3844, 105.0885) -> (186.7246, 104.4513)
  line L3218 (182.9166, 99.625) -> (183.129, 98.125)
  line L3219 (182.0837, 104.4376) -> (186.4224, 104.4376)
  line L3220 (187.3563, 105.2865) -> (186.4603, 106.2121)
  line L3221 (180.4262, 105.0875) -> (181.1762, 105.0875)
  line L3222 (188.1344, 105.0885) -> (187.3844, 105.0885)
  arc A473 (181.3511, 98.5549) -> (181.8462, 98.125) centre (181.8462, 98.625) ccw
  line L3223 (181.1478, 105.2875) -> (180.3978, 105.2875)
  line L3224 (185.4054, 112.25) -> (185.6178, 110.75)
  arc A474 (187.1812, 111.8201) -> (186.6861, 112.25) centre (186.6861, 111.75) ccw
  line L3225 (180.3978, 105.2875) -> (179.412, 112.25)
  line L3226 (181.3394, 110.75) -> (181.127, 112.25)
  line L3227 (187.1203, 112.25) -> (188.1063, 105.2865)
  line L3228 (181.3454, 105.2002) -> (182.0837, 104.4376)
  line L3229 (180.927, 112.25) -> (181.8208, 105.9374)
  line L3230 (187.186, 105.1749) -> (186.4477, 105.9376)
  line L3231 (186.4603, 106.2121) -> (185.6054, 112.25)
  line L3232 (181.127, 112.25) -> (185.4054, 112.25)
  line L3233 (186.4477, 105.9376) -> (182.1089, 105.9376)
  line L3234 (185.6054, 112.25) -> (187.1203, 112.25)
  line L3235 (181.8208, 105.9374) -> (181.1478, 105.2875)
  line L3236 (198.3258, 110.75) -> (194.0474, 110.75)
  line L3237 (193.635, 112.25) -> (192.12, 112.25)
  arc A475 (201.2525, 98.125) -> (201.7476, 98.6951) centre (201.2525, 98.625) ccw
  circle A476 centre (192.12, 99) radius 0.875
  line L3238 (193.8842, 105.0875) -> (194.7802, 104.1619)
  line L3239 (200.3283, 98.125) -> (201.8283, 98.125)
  line L3240 (199.9139, 99.625) -> (195.6246, 99.625)
  line L3241 (194.8169, 105.9376) -> (194.0534, 105.2002)
  line L3242 (195.635, 98.125) -> (194.12, 98.125)
  line L3243 (194.12, 98.125) -> (193.1342, 105.0875)
  line L3244 (199.4326, 104.4513) -> (200.3283, 98.125)
  line L3245 (200.1263, 98.125) -> (199.9139, 99.625)
  line L3246 (199.1304, 104.4376) -> (199.894, 105.1749)
  line L3247 (200.8143, 105.2865) -> (200.0643, 105.2865)
  line L3248 (201.8283, 98.125) -> (200.8424, 105.0885)
  arc A477 (192.6958, 112.25) -> (192.2007, 111.6799) centre (192.6958, 111.75) ccw
  line L3249 (195.837, 98.125) -> (200.1263, 98.125)
  line L3250 (194.7802, 104.1619) -> (195.635, 98.125)
  line L3251 (200.0924, 105.0885) -> (199.4326, 104.4513)
  line L3252 (195.6246, 99.625) -> (195.837, 98.125)
  line L3253 (194.7917, 104.4376) -> (199.1304, 104.4376)
  line L3254 (200.0643, 105.2865) -> (199.1683, 106.2121)
  line L3255 (193.1342, 105.0875) -> (193.8842, 105.0875)
  line L3256 (200.8424, 105.0885) -> (200.0924, 105.0885)
  arc A478 (194.0591, 98.5549) -> (194.5542, 98.125) centre (194.5542, 98.625) ccw
  line L3257 (193.8558, 105.2875) -> (193.1058, 105.2875)
  line L3258 (198.1134, 112.25) -> (198.3258, 110.75)
  arc A479 (199.8892, 111.8201) -> (199.3941, 112.25) centre (199.3941, 111.75) ccw
  line L3259 (193.1058, 105.2875) -> (192.12, 112.25)
  line L3260 (194.0474, 110.75) -> (193.835, 112.25)
  line L3261 (199.8283, 112.25) -> (200.8143, 105.2865)
  line L3262 (194.0534, 105.2002) -> (194.7917, 104.4376)
  line L3263 (193.635, 112.25) -> (194.5288, 105.9374)
  line L3264 (199.894, 105.1749) -> (199.1557, 105.9376)
  line L3265 (199.1683, 106.2121) -> (198.3134, 112.25)
  line L3266 (193.835, 112.25) -> (198.1134, 112.25)
  line L3267 (199.1557, 105.9376) -> (194.8169, 105.9376)
  line L3268 (198.3134, 112.25) -> (199.8283, 112.25)
  line L3269 (194.5288, 105.9374) -> (193.8558, 105.2875)
  dimension "d5" = 203.3333
  dimension "d6" = 12.7083
  dimension "d7" = 19.125
  dimension "d8" = 114.75
  dimension "d9" = 1.75
  dimension "d10" = 3.375
  dimension "d11" = 1.5
  dimension "d13" = 1.5
  dimension "d15" = 2.5
  dimension "d16" = 3.5
  dimension "d17" = 3.5
  dimension "d19" = 1.5
  dimension "d23" = 16.625
  dimension "d26" = 0.75
  dimension "d27" = 0.2
  dimension "d28" = 0.2
  dimension "d29" = 0.2
  dimension "d30" = 0.2
  dimension "d31" = 1.5
  dimension "d32" = 0.2
  dimension "d34" = 0.2
  dimension "d37" = 0.2
  dimension "d38" = 0.2
  dimension "d39" = 136
  dimension "d43" = 14.2659
  dimension "d44" = 7.0329
  dimension "d45" = 0.2
  dimension "d46" = 1.5
  dimension "d47" = 1
  dimension "d50" = 12.708
  dimension "d51" = 19.125
  constraint horizontal L0
  constraint vertical L1
  constraint horizontal L2
  constraint vertical L3
  constraint coincident L0.start L3.end
  constraint parallel L6 L9
  constraint parallel L8 L15
  constraint parallel L18 L33
  constraint parallel L15 L18
  constraint parallel L20 L22
  constraint parallel L17 L20
  constraint parallel L17 L36
  constraint parallel L23 L25
  constraint parallel L31 L34
  constraint parallel L35 L38
  constraint collinear L31 L38
  constraint collinear L6 L25
  constraint collinear L10 L14
  constraint collinear L14 L39
  constraint parallel L16 L19
  constraint equal L16 L19
  constraint equal L12 L14
  constraint equal L27 L29
  constraint equal L11 L13
  constraint equal L10 L11
  constraint equal L13 L39
  constraint equal L30 L39
  constraint equal L26 L28
  constraint collinear L24 L29
  constraint collinear L29 L30
  constraint parallel L23 L26
  constraint parallel L9 L11
  constraint horizontal L14
  constraint horizontal L29
  constraint parallel L12 L14
  constraint horizontal L16
  constraint parallel L32 L37
  constraint parallel L7 L21
  constraint horizontal L21
  constraint equal L31 L38
  constraint equal L32 L37
  constraint equal L7 L21
  constraint equal L21 L32
  constraint horizontal L37
  constraint equal L15 L20
  constraint tangent L6 A2
  constraint tangent L10 A2
  constraint tangent L39 A3
  constraint tangent L38 A3
  constraint tangent L30 A4
  constraint tangent L31 A4
  constraint equal A2 A3
  constraint coincident L24.end L25.start
  constraint tangent L24 A1
  constraint tangent L25 A1
  constraint equal L6 L25
  constraint equal L11 L26
  constraint equal A1 A4
  constraint equal A3 A4
  constraint coincident L25 A1.end
  constraint coincident L24 A1.start
  constraint coincident L10 A2.end
  constraint coincident L6 A2.start
  constraint coincident L38 A3.end
  constraint coincident L39 A3.start
  constraint coincident L30 A4.end
  constraint coincident L31 A4.start
  measures "d5" distance of L0.start L4.end
  measures "d6" distance of L0.start L0.end
  measures "d7" distance of L0.start L2.end
  measures "d8" distance of L0.start L5.start
  measures "d9" diameter of A0
  measures "d10" vertical distance of L0.start A0.centre
  measures "d11" horizontal distance of L0.start A0.centre
  measures "d13" distance of L3 L38.end
  measures "d15" distance of L0 L28.end
  measures "d16" distance of L3 L30.end
  measures "d17" distance of L1 L6.start
  measures "d19" vertical distance of L11.start L11.end
  measures "d23" distance of L0 L10
  measures "d26" horizontal distance of L31.end L32.end
  measures "d27" distance of L20 L22
  measures "d28" distance of L8 L15
  measures "d29" distance of L18 L33
  measures "d30" distance of L17 L36
  measures "d31" distance of L16 L19
  measures "d32" distance of L23 L26
  measures "d34" distance of L28 L34
  measures "d37" distance of L9.end L11.start
  measures "d38" distance of L13.end L35.start
  measures "d39" angle of L21 L22
  measures "d43" distance of L6.start L24.end
  measures "d44" distance of L21.start L24.end
  measures "d45" distance of L32 L37
  measures "d46" distance of L23.end L24.end
  measures "d47" diameter of A1